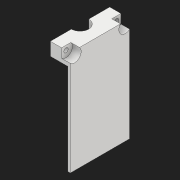
# Autodesk Inventor part: BP008
Saved by Autodesk Inventor 2017 SP1 (Build 210196100, 196)
## iProperties
Created: 2018-03-10
Part Number: BP008
Material: ABS Plastic
Document SubType Name: Modeling
Designer: Zach
Density: 1.06 g/cm^3
Appearance: CR White
Author: Zach
Autodesk Inventor part; units mm, degrees
ref_plane "YZ Plane" through (0, 0, 0) normal (1, 0, 0) x (0, 1, 0)
ref_plane "XZ Plane" through (0, 0, 0) normal (0, 1, 0) x (-1, 0, 0)
ref_plane "XY Plane" through (0, 0, 0) normal (0, 0, 1) x (1, 0, 0)
sketch "Sketch1" plane through (0, 0, 0) normal (0, 0, 1) x (1, 0, 0)
  circle A0 centre (-20, 34.2) radius 10 construction
  line L0 (0, 0) -> (0, 68.4)
  line L1 (0, 0) -> (-20, 0)
  line L2 (-20, 0) -> (-20, 68.4) construction
  line L3 (-20, 68.4) -> (0, 68.4)
  line L4 (-20, 68.4) -> (-20, 44.2)
  line L5 (-20, 0) -> (-20, 24.2)
  arc A1 (-20, 24.2) -> (-20, 44.2) centre (-20, 34.2) ccw
  point P0 (0, 34.2)
  dimension "d0" = 20
  dimension "d1" = 20
  dimension "d3" = 68.4
  constraints: 12 end point, 4 point on circle, 2 centre point, 2 horizontal, 2 midpoint, 2 point on line, 1 coincident, 1 concentric, 1 horizontal alignment, 1 perpendicular, 1 vertical
  measures "d0" diameter of A0
  measures "d1" distance from line of L0 A0.centre
  measures "d3" distance of L0.start L0.end
extrude "Extrusion1" add sketch "Sketch1" along normal blind 15
sketch "Sketch2" plane through (0, 0, 0) normal (1, 0, 0) x (0, 0, -1)
  line L0 (-15, 68.4) -> (-15, 44.2) projected
  line L1 (-15, 68.4) -> (105, 68.4)
  line L2 (105, 68.4) -> (105, 0)
  line L3 (105, 0) -> (-15, 0)
  line L4 (-15, 0) -> (-15, 68.4)
  point P0 (0, 0)
  dimension "d6" = 120
  constraints: 8 end point, 2 parallel, 1 horizontal, 1 perpendicular, 1 point on line
  measures "d6" distance of L2.end L3.end
extrude "Extrusion2" add sketch "Sketch2" along normal blind 3
sketch "Sketch3" plane through (-20, 0, 0) normal (-1, 0, 0) x (0, 0, 1)
  circle A0 centre (10, 5) radius 2.5
  circle A1 centre (10, 63.4) radius 2.5
  line L0 (0, 0) -> (15, 0) projected
  line L1 (15, 24.2) -> (15, 0) projected
  line L2 (15, 68.4) -> (15, 44.2) projected
  line L3 (0, 68.4) -> (15, 68.4) projected
  dimension "d9" = 5
  dimension "d10" = 5
  dimension "d11" = 5
  dimension "d12" = 5
  dimension "d13" = 5
  dimension "d14" = 5
  constraints: 2 centre point
  measures "d9" diameter of A0
  measures "d10" diameter of A1
  measures "d11" distance from line of L2 A1.centre
  measures "d12" distance from line of L3 A1.centre
  measures "d13" distance from line of A0.centre L1
  measures "d14" distance from line of L0 A0.centre
extrude "Extrusion3" cut sketch "Sketch3" against normal through all
sketch "Sketch4" plane through (3, 0, 0) normal (1, 0, 0) x (0, 0, -1)
  circle A0 centre (-10, 63.4) radius 2.5 projected
  circle A1 centre (-10, 5) radius 2.5 projected
  circle A2 centre (-10, 63.4) radius 2.5 projected
  circle A3 centre (-10, 63.4) radius 7.5
  circle A4 centre (-10, 5) radius 7.5
  point P0 (0, 0)
  dimension "d18" = 15
  dimension "d19" = 15
  constraints: 2 centre point, 2 coincident
  measures "d18" diameter of A3
  measures "d19" diameter of A4
extrude "Extrusion4" cut sketch "Sketch4" against normal blind 10 contours A0 | A1 | A3 | A4
body "Solid1"
